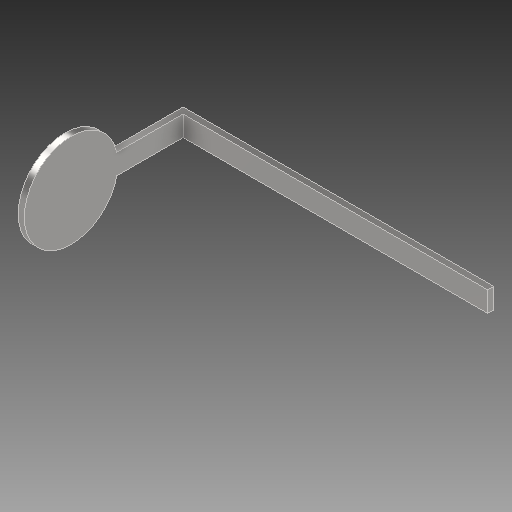
# Autodesk Inventor part: Mirror_ыефтв
Saved by Autodesk Inventor 2023 (Build 270158000, 158)
## iProperties
Created: 2022-01-17
Part Number: Mirror_ыефтв
Material: Сталь, мягкая
Document SubType Name: Modeling
Designer: Администратор
Density: 7.85 g/cm^3
Appearance: С умеренной полировкой
Mass: 108.19 g
Surface Area: 43.4318 cm^2
Volume: 13.7822 cm^3
Author: Администратор
Autodesk Inventor part; units mm, degrees
ref_plane "YZ Plane" through (0, 0, 0) normal (1, 0, 0) x (0, 1, 0)
ref_plane "XZ Plane" through (0, 0, 0) normal (0, 1, 0) x (-1, 0, 0)
ref_plane "XY Plane" through (0, 0, 0) normal (0, 0, 1) x (1, 0, 0)
sketch "Эскиз5" plane through (0, 0, 0) normal (0, 1, 0) x (-1, 0, 0)
  line L0 (152.615, 60) -> (152.615, -3)
  line L1 (152.615, -3) -> (0, -3)
  line L2 (0, -3) -> (0, 0)
  line L3 (0, 0) -> (149.615, 0)
  line L4 (149.615, 0) -> (149.615, 60)
  line L5 (149.615, 60) -> (152.615, 60)
  dimension "d40" = 149.615
  dimension "d41" = 3
  dimension "d42" = 60
  constraints: 12 end point, 6 perpendicular, 1 coincident, 1 vertical
  measures "d40" distance of L2.end L3.end
  measures "d41" distance of L4.end L0.start
  measures "d42" distance of L3.end L4.end
extrude "Выдавливание2" add sketch "Эскиз5" along normal blind 10
sketch "Эскиз6" plane through (-149.615, 0, 60) normal (1, 0, 0) x (0, 0, -1)
  line L0 (63, 0) -> (0, 0) projected
  line L1 (0, 10) -> (10, 10) construction
  line L2 (10, 10) -> (10, 0) construction
  line L3 (10, 0) -> (0, 0) construction
  line L4 (0, 0) -> (0, 10) construction
  line L5 (0, 10) -> (10, 0) construction
  line L6 (10, 10) -> (0, 0) construction
  circle A0 centre (5, 5) radius 23
  point P0 (60, 0)
  dimension "d45" = 46
  constraints: 12 end point, 3 perpendicular, 2 parallel, 1 centre point, 1 horizontal, 1 midpoint
  measures "d45" diameter of A0
extrude "Выдавливание3" add sketch "Эскиз6" against normal blind 3
